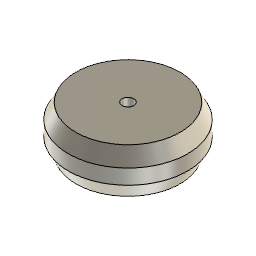
50.8mm TPU Wheel (Autodesk Fusion 360 design; units mm, degrees)
Autodesk Fusion 360 part; units mm, degrees
note: some values were not read from the file. Set by a fixed rule: which sketch regions a step uses.
sketch "Sketch1" plane through (0, 0, 0) normal (0, 0, 1) x (1, 0, 0)
  circle A0 centre (0, 0) radius 16.95
  circle A1 centre (0, 0) radius 14.605
  line L0 (0, 14.605) -> (-13.8902, 4.5132)
  line L1 (-13.8902, 4.5132) -> (-8.5846, -11.8157)
  line L2 (-8.5846, -11.8157) -> (8.5846, -11.8157)
  line L3 (8.5846, -11.8157) -> (13.8902, 4.5132)
  line L4 (13.8902, 4.5132) -> (0, 14.605)
  line L5 (0, 0) -> (0, 14.605)
  line L6 (0, 0) -> (-13.8902, 4.5132)
  line L7 (0, 0) -> (13.8902, 4.5132)
  line L8 (0, 0) -> (8.5846, -11.8157)
  line L9 (0, 0) -> (-8.5846, -11.8157)
  line L10 (0, 16.95) -> (-16.1204, 5.2378)
  line L11 (-16.1204, 5.2378) -> (-9.963, -13.7128)
  line L12 (-9.963, -13.7128) -> (9.963, -13.7128)
  line L13 (9.963, -13.7128) -> (16.1204, 5.2378)
  line L14 (16.1204, 5.2378) -> (0, 16.95)
  line L15 (0, 16.95) -> (0, 12.886)
  line L16 (16.1204, 5.2378) -> (12.2553, 3.982)
  line L17 (9.963, -13.7128) -> (7.5742, -10.425)
  line L18 (-9.963, -13.7128) -> (-7.5742, -10.425)
  line L19 (-16.1204, 5.2378) -> (-12.2553, 3.982)
  line L20 (-12.2553, 3.982) -> (-11.5242, 6.2322)
  line L21 (-12.2553, 3.982) -> (-12.9864, 1.7318)
  line L22 (-7.5742, -10.425) -> (-5.6601, -11.8157)
  line L23 (-7.5742, -10.425) -> (-9.4883, -9.0343)
  line L24 (7.5742, -10.425) -> (9.4883, -9.0343)
  line L25 (7.5742, -10.425) -> (5.6601, -11.8157)
  line L26 (12.2553, 3.982) -> (12.9864, 1.7318)
  line L27 (12.2553, 3.982) -> (11.5242, 6.2322)
  line L28 (0, 12.886) -> (2.366, 12.886)
  line L29 (0, 12.886) -> (-2.366, 12.886)
  circle A2 centre (0, 0) radius 6.985
  line L30 (0, -6.985) -> (6.6431, -2.1585)
  line L31 (6.6431, -2.1585) -> (4.1057, 5.651)
  line L32 (4.1057, 5.651) -> (-4.1057, 5.651)
  line L33 (-4.1057, 5.651) -> (-6.6431, -2.1585)
  line L34 (-6.6431, -2.1585) -> (0, -6.985)
  line L35 (0, -6.985) -> (-5.6601, -11.8157)
  line L36 (0, -6.985) -> (5.6601, -11.8157)
  line L37 (6.6431, -2.1585) -> (9.4883, -9.0343)
  line L38 (6.6431, -2.1585) -> (12.9864, 1.7318)
  line L39 (11.5242, 6.2322) -> (4.1057, 5.651)
  line L40 (4.1057, 5.651) -> (2.366, 12.886)
  line L41 (-2.366, 12.886) -> (-4.1057, 5.651)
  line L42 (-6.6431, -2.1585) -> (-9.4883, -9.0343)
  line L43 (-6.6431, -2.1585) -> (-12.9864, 1.7318)
  line L44 (-11.5242, 6.2322) -> (-4.1057, 5.651)
  line L45 (-12.9864, 1.7318) -> (-14.5949, 0.5428)
  line L46 (-11.5242, 6.2322) -> (-12.1266, 8.1395)
  line L47 (-2.366, 12.886) -> (-3.9938, 14.0483)
  line L48 (2.366, 12.886) -> (3.9938, 14.0483)
  line L49 (11.5242, 6.2322) -> (12.1266, 8.1395)
  line L50 (12.9864, 1.7318) -> (14.5949, 0.5428)
  line L51 (9.4883, -9.0343) -> (11.4885, -9.0178)
  line L52 (5.6601, -11.8157) -> (5.0263, -13.7128)
  line L53 (-5.6601, -11.8157) -> (-5.0263, -13.7128)
  line L54 (-9.4883, -9.0343) -> (-11.4885, -9.0178)
  circle A3 centre (0, 0) radius 22.225
  circle A4 centre (0, 0) radius 25.4
  dimension "d1" = 33.9
  dimension "d2" = 29.21
  dimension "d3" = 4.064
  dimension "d4" = 4.064
  dimension "d5" = 4.064
  dimension "d6" = 4.064
  dimension "d7" = 4.064
  dimension "d10" = 13.97
  dimension "d13" = 44.45
  dimension "d34" = 50.8
  constraint coincident A0.centre A1.centre
  constraint coincident A1 L0.start
  constraint vertical L5
  constraint coincident A0 L10.start
  constraint parallel L5 L15
  constraint parallel L7 L16
  constraint parallel L8 L17
  constraint parallel L9 L18
  constraint parallel L6 L19
  constraint coincident L0 L20.end
  constraint perpendicular L6 L20
  constraint coincident L1 L21.end
  constraint perpendicular L6 L21
  constraint coincident L2 L22.end
  constraint perpendicular L18 L22
  constraint coincident L1 L23.end
  constraint perpendicular L18 L23
  constraint coincident L3 L24.end
  constraint perpendicular L17 L24
  constraint coincident L2 L25.end
  constraint perpendicular L8 L25
  constraint coincident L3 L26.end
  constraint perpendicular L7 L26
  constraint coincident L4 L27.end
  constraint perpendicular L16 L27
  constraint coincident L4 L28.end
  constraint perpendicular L5 L28
  constraint coincident L0 L29.end
  constraint perpendicular L5 L29
  constraint concentric A0 A2
  constraint coincident A2 L30.start
  constraint coincident L11 L45.end
  constraint coincident A1 L45.end
  constraint coincident A1 L46.end
  constraint coincident L10 L46.end
  constraint coincident L10 L47.end
  constraint coincident A1 L47.end
  constraint coincident L14 L48.end
  constraint coincident A1 L48.end
  constraint coincident A1 L49.end
  constraint coincident L14 L49.end
  constraint coincident L13 L50.end
  constraint coincident A1 L50.end
  constraint coincident L13 L51.end
  constraint coincident A1 L51.end
  constraint coincident A1 L52.end
  constraint coincident L12 L52.end
  constraint coincident L12 L53.end
  constraint coincident A1 L53.end
  constraint coincident A1 L54.end
  constraint coincident L11 L54.end
  constraint concentric A2 A4
  measures "d1" diameter of A0
  measures "d2" diameter of A1
  measures "d3" distance of L10.start L15.end
  measures "d4" distance of L13.end L16.end
  measures "d5" distance of L12.end L17.end
  measures "d6" distance of L11.end L18.end
  measures "d7" distance of L10.end L19.end
  measures "d10" diameter of A2
  measures "d13" diameter of A3
  measures "d34" diameter of A4
extrude "Extrude1" add sketch "Sketch1" along normal blind 19.05 contours A0 A1 L13 | A0 A1 L14 | A1 L14 L16 | A1 L13 L16 | A0 A1 L12 | A1 L13 L17 | A1 L12 L17 | A0 A1 L10 | A1 L10 L15 | A1 L14 L15 | A1 L3 L50 | A1 L13 | L3 L13 L50 L51 | A1 L14 | L4 L14 L48 L49 | A1 L4 L49 | L4 L7 L16 L27 | L3 L7 L16 L26 | A0 A1 L11 | A1 L12 L18 | A1 L11 L18 | A1 L2 L52 | A1 L12 | L2 L12 L52 L53 | A1 L3 L51 | L3 L8 L17 L24 | L2 L8 L17 L25 | A1 L11 L19 | A1 L10 L19 | A1 L10 | L0 L10 L46 L47 | A1 L0 L47 | A1 L4 L48 | L0 L5 L15 L29 | L4 L5 L15 L28 | L7 L26 A2 L38 | L3 L37 L38 | L4 L39 L40 | L7 L27 A2 L39 | A1 L1 L54 | A1 L11 | L1 L11 L45 L54 | A1 L2 L53 | L2 L9 L18 L22 | L1 L9 L18 L23 | L8 L25 A2 L36 | L2 L35 L36 | L8 L24 A2 L37 | A1 L0 L46 | A1 L1 L45 | L1 L6 L19 L21 | L0 L6 L19 L20 | L0 L41 L44 | L5 L29 A2 L41 | L5 L28 A2 L40 | L7 A2 L31 | L8 A2 L30 | L7 L8 L30 L31 | L5 A2 L32 | L7 A2 L31 | L5 L7 L31 L32 | L9 L23 A2 L42 | L1 L42 L43 | L9 L22 A2 L35 | L8 A2 L30 | L8 L9 L30 L34 | L9 A2 L34 | L6 L20 A2 L44 | L6 L21 A2 L43 | L6 A2 L33 | L5 A2 L32 | L5 L6 L32 L33 | L9 A2 L34 | L6 A2 L33 | L6 L9 L33 L34 | A3 | A4
chamfer "Chamfer1" distance 3.175 distance2 6.35 1 edges at (-23.6811, -9.185, 19.05) measured on face at (1.8419, 7.6928, 19.05)
extrude "Extrude3" cut sketch "Sketch1" along normal blind 9.525 contours A0 A1 L13 | A0 A1 L14 | A1 L14 L16 | A1 L13 L16 | A0 A1 L12 | A1 L13 L17 | A1 L12 L17 | A0 A1 L10 | A1 L10 L15 | A1 L14 L15 | A1 L3 L50 | A1 L13 | L3 L13 L50 L51 | A1 L14 | L4 L14 L48 L49 | A1 L4 L49 | L4 L7 L16 L27 | L3 L7 L16 L26 | A0 A1 L11 | A1 L12 L18 | A1 L11 L18 | A1 L2 L52 | A1 L12 | L2 L12 L52 L53 | A1 L3 L51 | L3 L8 L17 L24 | L2 L8 L17 L25 | A1 L11 L19 | A1 L10 L19 | A1 L10 | L0 L10 L46 L47 | A1 L0 L47 | A1 L4 L48 | L0 L5 L15 L29 | L4 L5 L15 L28 | L7 L26 A2 L38 | L3 L37 L38 | L4 L39 L40 | L7 L27 A2 L39 | A1 L1 L54 | A1 L11 | L1 L11 L45 L54 | A1 L2 L53 | L2 L9 L18 L22 | L1 L9 L18 L23 | L8 L25 A2 L36 | L2 L35 L36 | L8 L24 A2 L37 | A1 L0 L46 | A1 L1 L45 | L1 L6 L19 L21 | L0 L6 L19 L20 | L0 L41 L44 | L5 L29 A2 L41 | L5 L28 A2 L40 | L7 A2 L31 | L8 A2 L30 | L7 L8 L30 L31 | L5 A2 L32 | L7 A2 L31 | L5 L7 L31 L32 | L9 L23 A2 L42 | L1 L42 L43 | L9 L22 A2 L35 | L8 A2 L30 | L8 L9 L30 L34 | L9 A2 L34 | L6 L20 A2 L44 | L6 L21 A2 L43 | L6 A2 L33 | L5 A2 L32 | L5 L6 L32 L33 | L9 A2 L34 | L6 A2 L33 | L6 L9 L33 L34
fillet "Fillet1" radius 2.54 1 edges at (-15.8029, -6.1294, 9.525)
extrude "Extrude4" add sketch "Sketch1" against normal blind 3.81 from surface at 9.525 contours A1 L13 | L3 L13 L50 L51 | A1 L14 | L4 L14 L48 L49 | A1 L12 | L2 L12 L52 L53 | A1 L10 | L0 L10 L46 L47 | L3 L37 L38 | L4 L39 L40 | A1 L11 | L1 L11 L45 L54 | L2 L35 L36 | L0 L41 L44 | L1 L42 L43
fillet "Fillet2" radius 1.27 20 edges at (5.0263, -13.7128, 7.6163) (-5.0263, -13.7128, 7.6163) (-5.6601, -11.8157, 7.62) (5.6601, -11.8157, 7.62) (-9.4883, -9.0343, 7.62) (-11.4885, -9.0178, 7.6163) (-14.5949, 0.5428, 7.6163) (-12.9864, 1.7318, 7.62) (-12.1266, 8.1395, 7.6163) (-11.5242, 6.2322, 7.62) (-2.366, 12.886, 7.62) (-3.9938, 14.0483, 7.6163) (2.366, 12.886, 7.62) (3.9938, 14.0483, 7.6163) (11.5242, 6.2322, 7.62) (12.1266, 8.1395, 7.6163) (13.7907, 1.1373, 5.715) (12.9864, 1.7318, 7.62) (11.4885, -9.0178, 7.6163) (9.4883, -9.0343, 7.62)
fillet "Fillet3" radius 2.54 5 edges at (-6.6431, -2.1585, 7.62) (-4.1057, 5.651, 7.62) (0, -6.985, 7.62) (6.6431, -2.1585, 7.62) (4.1057, 5.651, 7.62)
sketch "Sketch2" plane through (0, 0, 19.05) normal (0, 0, 1) x (-1, 0, 0)
  circle A0 centre (0, 0) radius 2.5
  circle A1 centre (0, 0) radius 22.225
  dimension "d31" = 5
  constraint coincident A0.centre A1.centre
  measures "d31" diameter of A0
extrude "Extrude5" cut sketch "Sketch2" against normal blind 9.525 contours A0
chamfer "Chamfer3" distance 6.35 distance2 3.175 1 edges at (-23.6811, -9.185, 0) measured on face at (25.2738, -2.529, 8.4667)
